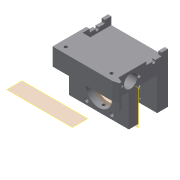
# Autodesk Inventor part: 01_Slide_camera_x_v0
Saved by Autodesk Inventor 2019.4 (Build 234330000, 330)
## iProperties
Created: 2020-10-27
Part Number: 01_Slide_camera_x_v0
Material: Generic
Document SubType Name: Modeling
Designer: diederichbenedict
Density: 1 g/cm^3
Appearance: Default
Author: diederichbenedict
Autodesk Inventor part; units mm, degrees
ref_plane "YZ Plane" through (0, 0, 0) normal (1, 0, 0) x (0, 1, 0)
ref_plane "XZ Plane" through (0, 0, 0) normal (0, 1, 0) x (-1, 0, 0)
ref_plane "XY Plane" through (0, 0, 0) normal (0, 0, 1) x (1, 0, 0)
ref_plane "Work Plane5" through (13.4046, 50.1721, 72.2727) normal (0, 1, 0) x (1, 0, 0)
sketch "Sketch7" plane through (13.4046, 50.1721, 72.2727) normal (0, 1, 0) x (1, 0, 0)
  circle A0 centre (6.5, 6.5) radius 2.5 construction
  circle A1 centre (48.5, 6.5) radius 2.5 construction
  line L0 (55, 2) -> (55, 11) construction
  line L1 (55, 35) -> (55, 44) construction
  circle A2 centre (48.5, 39.5) radius 2.5 construction
  circle A3 centre (6.5, 39.5) radius 2.5 construction
  line L2 (0, 35) -> (0, 44) construction
  line L3 (16.5, 85.8) -> (16.5, 84) construction
  line L4 (38.5, 85.8) -> (38.5, 84) construction
  line L5 (38.5, 84) -> (16.5, 84) construction
  line L6 (2, 0) -> (53, 0) construction
  line L7 (0, 38.8) -> (55, 38.8)
  line L8 (55, 38.8) -> (55, 85.8)
  line L9 (55, 85.8) -> (0, 85.8)
  line L10 (0, 85.8) -> (0, 38.8)
  line L11 (0, 85.8) -> (55, 85.8)
  line L12 (55, 85.8) -> (55, 89.8)
  line L13 (55, 89.8) -> (0, 89.8)
  line L14 (0, 89.8) -> (0, 85.8)
  point P0 (-13.4046, 72.2727)
  dimension "d112" = 47
  dimension "d115" = 4
  constraints: 30 end point, 5 vertical, 4 centre point, 4 horizontal, 4 parallel, 2 perpendicular, 1 point on line, 20 other
  measures "d112" distance between parallel lines of L7 L9
  measures "d115" distance of L12.end L11.end
extrude "Extrusion7" add sketch "Sketch7" along normal blind 16
sketch "Sketch8" plane through (13.4046, 50.1721, -13.5273) normal (-1, 0, 0) x (0, 0, 1)
  circle A0 centre (50.2042, 7.5) radius 2.3
  circle A1 centre (30.4132, 7.5) radius 6
  point P0 (13.5273, -50.1721)
  dimension "d77" = 12
  constraints: 2 centre point, 2 other
  measures "d77" diameter of A1
extrude "Extrusion8" cut sketch "Sketch8" against normal through all contours A1
sketch "Sketch9" plane through (13.4046, 50.1721, 72.2727) normal (0, -1, 0) x (1, 0, 0)
  circle A0 centre (48.5, -44.5) radius 2.5
  circle A1 centre (6.5, -44.5) radius 2.5
  ellipse E0 centre (6.4724, -21.5) end of major axis (6.4724, -19) minor radius 2.5
  ellipse E1 centre (48.4722, -21.5) end of major axis (48.4722, -19) minor radius 2.5
  point P0 (-13.4046, -72.2727)
  point P1 (6.5, -6.5)
  point P2 (48.5, -6.5)
  constraints: 2 centre point, 12 other
hole "Hole1" at (19.9046, 50.1721, 65.7727) at (61.9046, 50.1721, 65.7727) at (61.9046, 50.1721, 27.7727) at (19.9046, 50.1721, 27.7727) at (61.8768, 50.1721, 50.7727) at (19.877, 50.1721, 50.7727) direction (0, 1, 0) diameter 2.9 end through all
sketch "Sketch10" plane through (68.4046, 50.1721, -17.5273) normal (0, 0, -1) x (-1, 0, 0)
  circle A0 centre (39, -26) radius 1
  circle A1 centre (16, -26) radius 1
  circle A2 centre (16, -3) radius 1
  circle A3 centre (39, -3) radius 1.1
  circle A4 centre (27.5, -14.5) radius 12
  circle A5 centre (27.5, -14.5) radius 10.8
  line L0 (55, 0) -> (0, 0) projected
  line L1 (11.5, -29) -> (43.5, -29)
  line L2 (43.5, -29) -> (43.5, 0)
  line L3 (43.5, 0) -> (11.5, 0)
  line L4 (11.5, 0) -> (11.5, -29)
  line L5 (11.5, -29) -> (43.5, 0) construction
  line L6 (43.5, -29) -> (11.5, 0) construction
  line L7 (0, 0) -> (11.5, 0)
  line L8 (43.5, 0) -> (55, 0)
  line L9 (55, 0) -> (43.5, 0)
  line L10 (43.5, 0) -> (43.5, -29)
  line L11 (43.5, -29) -> (55, -29)
  line L12 (55, -29) -> (55, 0)
  line L13 (11.5, -29) -> (0, -29)
  line L14 (0, -29) -> (0, 0)
  line L15 (0, 0) -> (11.5, 0)
  line L16 (11.5, 0) -> (11.5, -29)
  circle A6 centre (47.5, -14.5) radius 3 construction
  circle A7 centre (7.5, -14.5) radius 3 construction
  circle A8 centre (47.5, -14.5) radius 3.1
  circle A9 centre (7.5, -14.5) radius 3.1
  line L17 (21.9985, -30) -> (32.9661, -30)
  line L18 (55, -29) -> (0, -29)
  line L19 (0, -29) -> (0, -30)
  line L20 (0, -30) -> (55, -30)
  line L21 (55, -30) -> (55, -29)
  point P0 (68.4046, -50.1721)
  dimension "d50" = 24
  dimension "d51" = 32
  dimension "d67" = 6.2
  dimension "d68" = 6.2
  constraints: 42 end point, 10 centre point, 8 parallel, 5 horizontal, 4 perpendicular, 2 coincident, 2 collinear, 2 midpoint, 1 point on line, 16 other
  measures "d50" diameter of A4
  measures "d51" distance of L3.end L2.end
  measures "d67" diameter of A8
  measures "d68" diameter of A9
extrude "Extrusion9" add sketch "Sketch10" against normal blind 10 contours L12 L11 L2 L0 | L2 L1 L4 L0 | L21 L20 L17 L19 L13 L1 L11 | L4 L13 L14 L0 | A8 | A9
sketch "Sketch15" plane through (68.4046, 50.1721, 33.4727) normal (1, 0, 0) x (0, 0, -1)
  line L0 (41, 0) -> (0, 0) projected
  line L1 (0, 16) -> (51, 16) projected
  line L2 (0, 0) -> (0, 16) projected
  line L3 (51, 16) -> (0, 16) projected
  line L4 (28, 16) -> (0, 16)
  line L5 (0, 16) -> (0, 7)
  line L6 (0, 7) -> (28, 7)
  line L7 (51, 9) -> (44.5, 9) construction
  line L8 (24.9, 18.4) -> (24.9, 10.6) construction
  line L9 (55.3238, 21.5045) -> (24.6, 21.5045)
  line L10 (24.6, 21.5045) -> (24.6, 8.9)
  line L11 (24.6, 8.9) -> (55.3238, 8.9)
  line L12 (55.3238, 8.9) -> (55.3238, 21.5045)
  line L13 (51, -30) -> (51, 16) projected
  line L14 (41, -30) -> (41, 0) projected
  line L15 (51, -30) -> (41, -30) projected
  point P0 (33.4727, -50.1721)
  point P1 (47, 16)
  dimension "d73" = 7
  dimension "d113" = 0.1
  dimension "d114" = 0.3
  constraints: 18 end point, 3 horizontal, 3 parallel, 2 perpendicular, 2 point on line, 1 vertical, 4 other
  measures "d73" distance between parallel lines of L6 L0
  measures "d113" distance from line of L7.start L11
  measures "d114" distance from line of L8.end L10
extrude "Extrusion12" cut sketch "Sketch15" against normal through all contours L13 L1 L10 L9 L12 L11 | L11 L10 L1 L13
sketch "Sketch17" plane through (13.4046, 50.1721, 72.2727) normal (0, -1, 0) x (1, 0, 0)
  circle A0 centre (37.5, -66.9) radius 1.5
  circle A1 centre (17.5, -66.9) radius 1.25
  circle A2 centre (17.5, -86.9) radius 1.25
  circle A3 centre (37.5, -86.9) radius 1.25
  point P0 (-13.4046, -72.2727)
  constraints: 4 centre point, 8 other
hole "Hole4" at (50.9046, 50.1721, 5.3727) at (30.9046, 50.1721, 5.3727) direction (0, 1, 0) diameter 3.5 end through all counterbore diameter 7 counterbore depth 4
ref_plane "Work Plane8" through (68.4046, 50.1721, 12.4727) normal (0, 0, 1) x (1, 0, 0)
sketch "Sketch18" plane through (68.4046, 50.1721, 12.4727) normal (0, 0, 1) x (1, 0, 0)
  circle A0 centre (-27.5, -14.5) radius 12 projected
  circle A1 centre (-39, -3) radius 1.1 projected
  circle A2 centre (-16, -3) radius 1 projected
  circle A3 centre (-16, -26) radius 1 projected
  circle A4 centre (-39, -26) radius 1 projected
  line L0 (0, -30) -> (0, 0) projected
  line L1 (-55, 0) -> (0, 0) projected
  line L2 (-55, 0) -> (-55, -30) projected
  line L3 (-55, -30) -> (0, -30) projected
  point P0 (-68.4046, -50.1721)
extrude "Extrusion13" add sketch "Sketch18" along normal blind 6 and the other way blind 3
sketch "Sketch23" plane through (13.4046, 50.1721, 33.4727) normal (-1, 0, 0) x (0, 0, 1)
  line L0 (-24.6, 8.9) -> (-51, 8.9) projected
  line L1 (-51, 8.9) -> (-51, -30) projected
  line L2 (-41, 0) -> (-41, -30) projected
  line L3 (-24, 0) -> (-41, 0) projected
  line L4 (0, 0) -> (0, 16) projected
  line L5 (-24.6, 16) -> (0, 16) projected
  line L6 (-24.6, 16) -> (-24.6, 8.9) projected
  circle A0 centre (-16.5868, 7.5) radius 6 projected
  line L7 (-24.6, 16) -> (-51, 16)
  line L8 (-51, 16) -> (-51, 8.9)
  line L9 (-51, 8.9) -> (-24.6, 8.9)
  line L10 (-24.6, 8.9) -> (-24.6, 16)
  line L11 (-31.1222, 16) -> (-45.0868, 16)
  line L12 (-45.0868, 16) -> (-45.0868, 13)
  line L13 (-45.0868, 13) -> (-31.1222, 13)
  line L14 (-31.1222, 13) -> (-31.1222, 16)
  line L15 (-32.6207, 14) -> (-43.5883, 14)
  line L16 (-32.1222, 15.1785) -> (-32.1221, 14.4985)
  line L17 (-43.5883, 14) -> (-44.0868, 14.4985)
  circle A1 centre (-31.2, 11.995) radius 2.1 construction
  circle A2 centre (-45, 11.995) radius 2.1 construction
  line L18 (-24, -30) -> (-24, 0) projected
  line L19 (-15, 0) -> (-15, -30) projected
  line L20 (0, 0) -> (-15, 0) projected
  line L21 (-51, -30) -> (-41, -30) projected
  line L22 (-15, -30) -> (-24, -30) projected
  point P0 (-33.4727, -50.1721)
  dimension "d116" = 1
  dimension "d117" = 1
  dimension "d118" = 1
  constraints: 22 end point, 4 parallel, 3 horizontal, 2 centre point, 2 perpendicular, 1 point on line, 11 other
  measures "d116" distance from line of L13 L15.end
  measures "d117" distance from line of L14 L16.start
  measures "d118" distance from line of L12 L17.end
extrude "Extrusion18" add sketch "Sketch23" against normal blind 3 contours L0 L8 L7 L12 L13 L14 L6
sketch "Sketch24" plane through (13.4046, 50.1721, 33.4727) normal (-1, 0, 0) x (0, 0, 1)
  circle A0 centre (-45, 11.995) radius 2.1
  circle A1 centre (-31.2, 11.995) radius 2.1
  circle A2 centre (-38.1, 11.995) radius 1.5
  point P0 (-33.4727, -50.1721)
  dimension "d121" = 3
  dimension "d122" = 6.9
  constraints: 3 centre point, 4 other
  measures "d121" diameter of A2
  measures "d122" distance of A2.centre A1.centre
extrude "Extrusion19" cut sketch "Sketch24" against normal through all contours A2
sketch "Sketch25" plane through (68.4046, 50.1721, 33.4727) normal (1, 0, 0) x (0, 0, -1)
  circle A0 centre (16.5868, 7.5) radius 6 projected
  arc A1 (36.9865, 13) -> (39.2136, 13) centre (38.1, 11.995) ccw projected
  line L0 (39.2136, 13) -> (45.0868, 13) projected
  line L1 (45.0868, 13) -> (45.0868, 16) projected
  line L2 (45.0868, 16) -> (51, 16) projected
  line L3 (51, 16) -> (51, -30) projected
  line L4 (41, 0) -> (41, -30) projected
  line L5 (24, 0) -> (41, 0) projected
  line L6 (0, 0) -> (0, 16) projected
  line L7 (31.1222, 16) -> (0, 16) projected
  line L8 (31.1222, 16) -> (31.1222, 13) projected
  line L9 (31.1222, 13) -> (36.9865, 13) projected
  line L10 (51, 8.9) -> (47.0344, 8.9) projected
  line L11 (51, 8.9) -> (24.5983, 8.9)
  line L12 (24.5983, 8.9) -> (24.5983, 16)
  line L13 (24, -30) -> (24, 0) projected
  line L14 (15, 0) -> (15, -30) projected
  line L15 (0, 0) -> (15, 0) projected
  line L16 (51, -30) -> (41, -30) projected
  line L17 (15, -30) -> (24, -30) projected
  point P0 (33.4727, -50.1721)
  constraints: 4 end point, 1 horizontal, 1 perpendicular, 1 point on line
extrude "Extrusion20" add sketch "Sketch25" against normal blind 3 contours A1 L0 L1 L2 L3 L10 L11 L12 L7 L8 L9
sketch "Sketch26" plane through (68.4046, 50.1721, 33.4727) normal (1, 0, 0) x (0, 0, -1)
  circle A0 centre (24.5868, 7.5) radius 1.625
  circle A1 centre (8.5868, 7.5) radius 1.625
  point P0 (33.4727, -50.1721)
  constraints: 2 centre point, 4 other
hole "Hole5" at (68.4046, 57.6721, 8.8859) at (68.4046, 57.6721, 24.8859) direction (-1, 0, 0) diameter 2.8 end through all
sketch "Sketch28" plane through (68.4046, 50.1721, 18.4727) normal (0, 0, 1) x (1, 0, 0)
  circle A0 centre (-27.5, -14.5) radius 12 projected
  circle A1 centre (-39, -3) radius 1.1 projected
  circle A2 centre (-39, -26) radius 1 projected
  circle A3 centre (-16, -26) radius 1 projected
  circle A4 centre (-16, -3) radius 1 projected
  line L0 (0, -30) -> (0, 0) projected
  line L1 (-55, 0) -> (0, 0) projected
  line L2 (-55, 0) -> (-55, -30) projected
  line L3 (-55, -30) -> (0, -30) projected
  point P0 (-68.4046, -50.1721)
hole "Hole7" at (52.4046, 24.1721, 18.4727) at (29.4046, 24.1721, 18.4727) at (29.4046, 47.1721, 18.4727) at (52.4046, 47.1721, 18.4727) direction (0, 0, -1) diameter 4 depth 8 tip angle 118
sketch "Sketch29" plane through (13.4046, 20.1721, -17.5273) normal (0, -1, 0) x (1, 0, 0)
  line L0 (0, 0) -> (55, 0) projected
  line L1 (55, 0) -> (55, 10) projected
  line L2 (0, 10) -> (55, 10) projected
  line L3 (0, 0) -> (0, 10) projected
  line L4 (55, 36) -> (55, 27) projected
  line L5 (0, 36) -> (55, 36) projected
  line L6 (0, 36) -> (0, 27) projected
  line L7 (55, 27) -> (0, 27) projected
  arc A0 (29.113, 42.4017) -> (29.113, 40.9628) centre (27.5177, 41.6823) ccw
  circle A1 centre (27.5177, 31.5) radius 1.4
  circle A2 centre (27.5177, 6.5) radius 1.4
  line L8 (50.0177, 6.5) -> (5.0177, 6.5)
  line L9 (5.0177, 6.5) -> (5.0177, 31.5)
  line L10 (5.0177, 31.5) -> (50.0177, 31.5)
  line L11 (50.0177, 31.5) -> (50.0177, 6.5)
  line L12 (50.0177, 6.5) -> (5.0177, 31.5) construction
  line L13 (5.0177, 6.5) -> (50.0177, 31.5) construction
  point P0 (-13.4046, 17.5273)
  point P1 (27.5177, 19)
  dimension "d150" = 2.8
  dimension "d151" = 2.8
  dimension "d152" = 45
  dimension "d153" = 25
  constraints: 12 end point, 4 midpoint, 3 centre point, 2 parallel, 2 point on circle, 1 horizontal, 1 perpendicular, 4 other
  measures "d150" diameter of A1
  measures "d151" diameter of A2
  measures "d152" distance of L9.end L10.end
  measures "d153" distance from line of A1.centre L8
hole "Hole8" at (18.4223, 20.1721, 13.9727) at (40.9223, 20.1721, 13.9727) at (63.4223, 20.1721, 13.9727) at (63.4223, 20.1721, -11.0273) at (40.9223, 20.1721, -11.0273) at (18.4223, 20.1721, -11.0273) direction (0, 1, 0) diameter 2.8 depth 8 tip angle 118
sketch "Sketch30" plane through (13.4046, 50.1721, 72.2727) normal (0, -1, 0) x (1, 0, 0)
  circle A0 centre (6.5, -44.5) radius 1.45 projected
  circle A1 centre (48.5, -44.5) radius 1.45 projected
  line L0 (0, -53.8) -> (55, -53.8) projected
  line L1 (55, -53.8) -> (55, -38.8) projected
  line L2 (0, -38.8) -> (55, -38.8) projected
  line L3 (0, -38.8) -> (0, -53.8) projected
  line L4 (55, -53.8) -> (55, -38.8) projected
  line L5 (55, -42.175) -> (60, -42.175)
  line L6 (60, -42.175) -> (60, -40.175)
  line L7 (60, -40.175) -> (55, -40.175)
  line L8 (55, -40.175) -> (55, -42.175)
  point P0 (-13.4046, -72.2727)
  dimension "d161" = 5
  dimension "d162" = 2
  constraints: 8 end point, 2 parallel, 1 horizontal, 1 perpendicular, 1 point on line
  measures "d161" distance of L7.end L6.end
  measures "d162" distance of L6.end L5.end
ref_plane "Work Plane9" through (67.562, 43.9221, 32.5482) normal (0, -1, 0) x (1, 0, 0)
extrude "Extrusion21" add sketch "Sketch30" against normal up to surface (22.25 mm away) from surface at 6.25 contours L1 L7 L6 L5
sketch "Sketch31" plane through (13.4046, 66.1721, 72.2727) normal (0, 1, 0) x (1, 0, 0)
  circle A0 centre (48.5, 44.5) radius 1.45 projected
  circle A1 centre (6.5, 44.5) radius 1.45 projected
  line L0 (55, 38.8) -> (55, 40.175) projected
  line L1 (60, 40.175) -> (55, 40.175) projected
  line L2 (60, 42.175) -> (60, 40.175) projected
  line L3 (55, 42.175) -> (60, 42.175) projected
  line L4 (55, 42.175) -> (55, 69.9222) projected
  line L5 (55, 69.9222) -> (52, 69.9222) construction
  line L6 (52, 63.4) -> (52, 69.9222) construction
  line L7 (52, 63.4) -> (3, 63.4) projected
  line L8 (3, 69.9222) -> (3, 63.4) projected
  line L9 (3, 69.9222) -> (0, 69.9222) projected
  line L10 (0, 69.9222) -> (0, 38.8) projected
  line L11 (0, 38.8) -> (55, 38.8) projected
  line L12 (60, 40.175) -> (55, 40.175) projected
  line L13 (0, 38.8) -> (55, 38.8) projected
  line L14 (60, 40.175) -> (55, 38.8)
  line L15 (55, 38.8) -> (55, 44.5)
  line L16 (55, 42.175) -> (60, 42.175) projected
  line L17 (60, 42.175) -> (55, 44.2246)
  point P0 (-13.4046, 72.2727)
  constraints: 6 end point, 2 point on line
ref_plane "Work Plane10" through (13.3602, 50.0901, 21.2671) normal (-0.0029789, 0.9999956, 0) x (0, 0, 1)
extrude "Extrusion22" add sketch "Sketch31" against normal up to surface contours L0 L1 L14 | L15 L3 L2 L1 | L4 L17 L3 surface through (13.3602, 50.0901, 21.2671) normal (-0.0029789, 0.9999956, 0)
body "Solid2"
